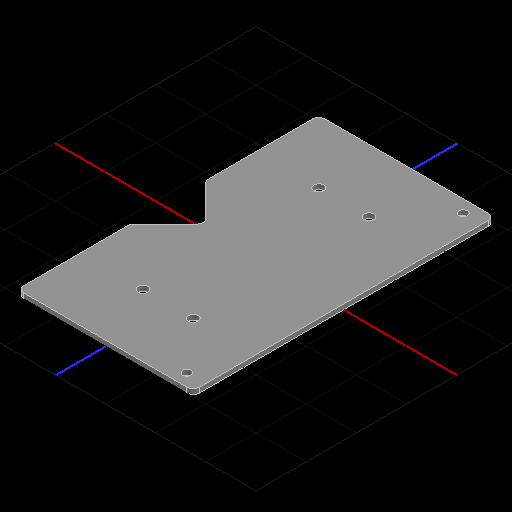
# Autodesk Inventor part: match_loader
Saved by Autodesk Inventor 2025.2 (Build 292293000, 293)
## iProperties
Created: 2025-12-09
Part Number: match_loader
Material: Generic
Document SubType Name: Modeling
Designer: cloudy
Density: 1 g/cm^3
Appearance: Smooth - Dark Gray
Author: cloudy
Autodesk Inventor part; units mm, degrees
ref_plane "YZ Plane" through (0, 0, 0) normal (1, 0, 0) x (0, 1, 0)
ref_plane "XZ Plane" through (0, 0, 0) normal (0, 1, 0) x (-1, 0, 0)
sketch "Sketch1" plane through (0, 0, 0) normal (0, 1, 0) x (-1, 0, 0)
  line L0 (44.45, 76.2) -> (-44.45, 76.2)
  line L1 (-44.45, -76.2) -> (44.45, -76.2)
  line L2 (44.45, 76.2) -> (-44.45, -76.2) construction
  line L3 (-44.45, 76.2) -> (44.45, -76.2) construction
  line L4 (0, 0) -> (-53.721, 0) construction
  line L5 (-44.45, 76.2) -> (-44.45, -76.2)
  line L6 (-44.45, -35.3838) -> (-44.45, -76.2)
  line L7 (44.45, 19.05) -> (25.4, 0)
  line L8 (25.4, 0) -> (44.45, -19.05)
  line L9 (44.45, -76.2) -> (44.45, -19.05)
  line L10 (44.45, 19.05) -> (44.45, 76.2)
  point P0 (-12.7, 0)
  point P1 (-44.45, 0)
  dimension "d0" = 88.9
  dimension "d1" = 152.4
  dimension "d4" = 12.7
  dimension "d27" = 90
  dimension "d29" = 19.05
  constraints: 22 end point, 5 parallel, 3 midpoint, 3 perpendicular, 2 horizontal, 2 point on line
  measures "d0" distance of L1.end L1.start
  measures "d1" distance of L0.end L1.start
  measures "d4" distance of L4.start point (-12.7, 0)
  measures "d27" angle of L8 L7
  measures "d29" horizontal distance of L7.start L7.end
extrude "Extrusion1" add sketch "Sketch1" along normal blind 2.54
ref_plane "Work Plane1" through (-44.45, 0, 69.85) normal (0, 0, 1) x (1, 0, 0)
sketch "Sketch3" plane through (0, 0, 0) normal (0, -1, 0) x (1, 0, 0)
  arc A0 (41.275, 69.85) -> (34.925, 76.2) centre (34.925, 69.85) ccw projected
  circle A1 centre (34.925, 69.85) radius 2.1844
  circle A2 centre (34.925, -69.85) radius 2.1844
  arc A3 (34.925, -76.2) -> (41.275, -69.85) centre (34.925, -69.85) ccw projected
  point P0 (0, 0)
  dimension "d22" = 4.3688
  dimension "d23" = 4.3688
  constraints: 2 centre point, 1 coincident, 1 concentric
  measures "d22" diameter of A1
  measures "d23" diameter of A2
extrude "Extrusion3" cut sketch "Sketch3" against normal through all
fillet "Fillet2" radius 3.175 3 edges at (-25.4, 1.27, 0) (-44.45, 1.27, -19.05) (-44.45, 1.27, 19.05)
fillet "Fillet3" radius 3.175 4 edges at (-44.45, 1.27, -76.2) (44.45, 1.27, -76.2) (44.45, 1.27, 76.2) (-44.45, 1.27, 76.2)
sketch "Sketch4" plane through (0, 0, 0) normal (0, -1, 0) x (1, 0, 0)
  circle A0 centre (-12.7, 44.45) radius 2.54
  circle A1 centre (12.7, 44.45) radius 2.54
  circle A2 centre (-12.7, -44.45) radius 2.54
  circle A3 centre (12.7, -44.45) radius 2.54
  line L0 (41.275, -76.2) -> (-41.275, -76.2) projected
  line L1 (0, -76.2) -> (0, 76.2) construction
  line L2 (-41.275, 76.2) -> (41.275, 76.2) projected
  line L3 (-12.7, -44.45) -> (-12.7, 44.45) construction
  arc A4 (-27.6451, -2.2451) -> (-27.6451, 2.2451) centre (-29.8901, 0) ccw projected
  line L4 (-26.7151, 0) -> (44.45, 0) construction
  line L5 (44.45, 73.025) -> (44.45, -73.025) projected
  point P0 (0, 0)
  dimension "d33" = 25.4
  dimension "d34" = 5.08
  dimension "d35" = 88.9
  constraints: 6 end point, 4 centre point, 3 equal radius, 3 midpoint, 1 point on circle, 1 vertical, 3 other
  measures "d33" distance of A1.centre L3.end
  measures "d34" diameter of A0
  measures "d35" distance of L3.start L3.end
extrude "Extrusion4" cut sketch "Sketch4" against normal through all
body "Solid1"
